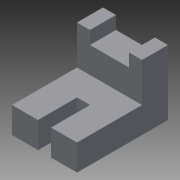
# Autodesk Inventor part: 4.1e Q3
Saved by Autodesk Inventor 2015 (Build 190159000, 159)
## iProperties
Created: 2017-11-15
Part Number: 4.1e Q3
Material: Generic
Document SubType Name: Modeling
Designer: Administrator
Density: 1 g/cm^3
Appearance: Default
Author: Administrator
Autodesk Inventor part; units mm, degrees
ref_plane "YZ Plane" through (0, 0, 0) normal (1, 0, 0) x (0, 1, 0)
ref_plane "XZ Plane" through (0, 0, 0) normal (0, 1, 0) x (-1, 0, 0)
ref_plane "XY Plane" through (0, 0, 0) normal (0, 0, 1) x (1, 0, 0)
sketch "Sketch1" plane through (0, 0, 0) normal (1, 0, 0) x (0, 1, 0)
  line L0 (0, 0) -> (25.4, 0)
  line L1 (25.4, 0) -> (25.4, -63.5)
  line L2 (25.4, -63.5) -> (63.5, -63.5)
  line L3 (63.5, -63.5) -> (63.5, -88.9)
  line L4 (63.5, -88.9) -> (0, -88.9)
  line L5 (0, -88.9) -> (0, 0)
  dimension "d0" = 25.4
  dimension "d1" = 25.4
  dimension "d2" = 88.9
  dimension "d3" = 63.5
  constraints: 12 end point, 5 perpendicular, 1 horizontal
  measures "d0" distance of L0.start L0.end
  measures "d1" distance of L2.end L3.end
  measures "d2" distance of L4.end L0.start
  measures "d3" distance of L3.end L4.end
extrude "Extrusion1" add sketch "Sketch1" along normal blind 63.5
sketch "Sketch2" plane through (0, 25.4, -63.5) normal (0, 0, 1) x (1, 0, 0)
  line L0 (0, 38.1) -> (63.5, 38.1) projected
  line L1 (12.7, 38.1) -> (12.7, 25.4)
  line L2 (12.7, 25.4) -> (50.8, 25.4)
  line L3 (50.8, 25.4) -> (50.8, 38.1)
  point P0 (0, -25.4)
  dimension "d6" = 12.7
  dimension "d7" = 38.1
  constraints: 6 end point, 2 perpendicular, 2 point on line, 1 vertical
  measures "d6" distance of L1.start L1.end
  measures "d7" distance of L1.end L2.end
extrude "Extrusion2" cut sketch "Sketch2" against normal blind 39.6875
sketch "Sketch3" plane through (0, 0, 0) normal (0, 0, 1) x (1, 0, 0)
  line L0 (0, 25.4) -> (63.5, 25.4) projected
  line L1 (25.4, 25.4) -> (25.4, 0)
  line L2 (25.4, 0) -> (38.1, 0)
  line L3 (38.1, 0) -> (38.1, 25.4)
  point P0 (0, 0)
  dimension "d10" = 25.4
  dimension "d11" = 12.7
  constraints: 6 end point, 2 point on line, 1 perpendicular, 1 vertical
  measures "d10" distance of L1.start L1.end
  measures "d11" distance of L1.end L2.end
extrude "Extrusion3" cut sketch "Sketch3" against normal blind 38.1
body "Solid1"
